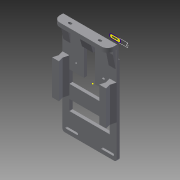
# Autodesk Inventor part: latte_d435_frame_s2new
Saved by Autodesk Inventor 2015 (Build 190159000, 159)
## iProperties
Created: 2021-11-17
Part Number: latte_d435_frame_s2new
Material: 常规
Document SubType Name: Modeling
Designer: chenhan
Density: 1 g/cm^3
Appearance: 默认
Author: chenhan
Autodesk Inventor part; units mm, degrees
ref_plane "YZ Plane" through (0, 0, 0) normal (1, 0, 0) x (0, 1, 0)
ref_plane "XZ Plane" through (0, 0, 0) normal (0, 1, 0) x (-1, 0, 0)
ref_plane "XY Plane" through (0, 0, 0) normal (0, 0, 1) x (1, 0, 0)
sketch "草图1" plane through (0, 0, 0) normal (0, 1, 0) x (-1, 0, 0)
  circle A0 centre (0, -42.5) radius 3.2
  circle A1 centre (0, -42.5) radius 1.6
  line L0 (63, 0) -> (-63, 0) projected
  circle A2 centre (19.7, 18.67) radius 1.6
  line L1 (0, -107.6) -> (0, 110.1) projected
  circle A3 centre (0, 42.5) radius 3.2
  circle A4 centre (0, 42.5) radius 1.6
  line L2 (-19.7, 18.67) -> (-19.7, -30.5269)
  line L3 (-19.7, -5.9284) -> (-19.7, -9.9284) construction
  line L4 (-20.95, -5.9284) -> (-20.95, -9.9284)
  line L5 (-18.45, -9.9284) -> (-18.45, -5.9284)
  arc A5 (-18.45, -5.9284) -> (-20.95, -5.9284) centre (-19.7, -5.9284) ccw
  arc A6 (-20.95, -9.9284) -> (-18.45, -9.9284) centre (-19.7, -9.9284) ccw
  line L6 (-22.2311, 18.67) -> (-17.1689, 18.67) construction
  line L7 (-18.7, 18.67) -> (-20.7, 18.67) construction
  line L8 (-18.7, 19.92) -> (-20.7, 19.92)
  line L9 (-20.7, 17.42) -> (-18.7, 17.42)
  arc A7 (-18.7, 17.42) -> (-18.7, 19.92) centre (-18.7, 18.67) ccw
  arc A8 (-20.7, 19.92) -> (-20.7, 17.42) centre (-20.7, 18.67) ccw
  line L10 (45, 79) -> (-45, 79)
  line L11 (-45, 79) -> (-45, 61.78)
  line L12 (-39, -76.5) -> (45, -76.5)
  line L13 (45, 61.78) -> (45, 79)
  line L14 (-39, 61.78) -> (-39, -76.5)
  line L15 (38, 73) -> (27.1169, 73)
  line L16 (39, 61.78) -> (45, 61.78)
  line L17 (-39, 61.78) -> (-45, 61.78)
  line L18 (37.25, 73) -> (27.25, 73) construction
  line L19 (37.25, 74.65) -> (27.25, 74.65)
  line L20 (27.25, 71.35) -> (37.25, 71.35)
  arc A9 (37.25, 71.35) -> (37.25, 74.65) centre (37.25, 73) ccw
  arc A10 (27.25, 74.65) -> (27.25, 71.35) centre (27.25, 73) ccw
  line L21 (34, -69.5) -> (18, -69.5) construction
  line L22 (34, -68) -> (18, -68)
  line L23 (18, -71) -> (34, -71)
  arc A11 (34, -71) -> (34, -68) centre (34, -69.5) ccw
  arc A12 (18, -68) -> (18, -71) centre (18, -69.5) ccw
  line L24 (-38, 73) -> (-27.1169, 73)
  line L25 (-37.25, 73) -> (-27.25, 73) construction
  line L26 (-37.25, 74.65) -> (-27.25, 74.65)
  line L27 (-27.25, 71.35) -> (-37.25, 71.35)
  arc A13 (-37.25, 74.65) -> (-37.25, 71.35) centre (-37.25, 73) ccw
  arc A14 (-27.25, 71.35) -> (-27.25, 74.65) centre (-27.25, 73) ccw
  line L28 (-34, -69.5) -> (-18, -69.5) construction
  line L29 (-34, -68) -> (-18, -68)
  line L30 (-18, -71) -> (-34, -71)
  arc A15 (-34, -68) -> (-34, -71) centre (-34, -69.5) ccw
  arc A16 (-18, -71) -> (-18, -68) centre (-18, -69.5) ccw
  line L31 (39, -27) -> (29, -27)
  line L32 (29, -27) -> (29, 23)
  line L33 (29, 23) -> (39, 23)
  line L34 (39, -27) -> (39, -27)
  line L35 (39, -27) -> (39, 31.5)
  line L36 (39, 31.5) -> (38.6344, 31.5)
  line L37 (39, 61.78) -> (39, 23)
  line L38 (39, -27) -> (39, -76.5)
  line L39 (39, -27) -> (29, -27)
  line L40 (29, -27) -> (29, 23)
  line L41 (29, 23) -> (39, 23)
  line L42 (39, 23) -> (39, -27)
  point P0 (0, 0)
  point P1 (-19.7, -7.9284)
  point P2 (32.25, 73)
  point P3 (26, -69.5)
  point P4 (-32.25, 73)
  point P5 (-26, -69.5)
  dimension "d0" = 6.4
  dimension "d1" = 3.2
  dimension "d2" = 42.5
  dimension "d7" = 3.2
  dimension "d8" = 19.7
  dimension "d9" = 18.67
  dimension "d10" = 4
  dimension "d14" = 2
  dimension "d15" = 2.5
  dimension "d16" = 39.4
  dimension "d18" = 90
  dimension "d20" = 45
  dimension "d23" = 3.3
  dimension "d24" = 32.25
  dimension "d25" = 10
  dimension "d27" = 16
  dimension "d28" = 3
  dimension "d30" = 26
  dimension "d56" = 106
  dimension "d57" = 50
  dimension "d67" = 10
  dimension "d85" = 2.5
  dimension "d86" = 4.35
  dimension "d127" = 79
  constraints: 95 end point, 24 point on circle, 19 symmetric about line, 17 centre point, 16 tangent, 10 parallel, 8 horizontal, 8 point on line, 7 perpendicular, 6 midpoint, 3 coincident, 2 vertical, 1 collinear, 6 other
  measures "d0" diameter of A0
  measures "d1" diameter of A1
  measures "d2" distance of point (0, 0) A0.centre
  measures "d7" diameter of A2
  measures "d8" horizontal distance of point (0, 0) A2.centre
  measures "d9" distance from line of L0 A2.centre
  measures "d10" distance of L3.start L3.end
  measures "d14" distance of L7.start L7.end
  measures "d15" diameter of A8
  measures "d16" distance from line of A2.centre L2
  measures "d18" distance of L10.start L10.end
  measures "d20" distance between parallel lines of L1 L13
  measures "d23" diameter of A10
  measures "d24" distance from line of L1 point (32.25, 73)
  measures "d25" distance of L18.end L18.start
  measures "d27" distance of L21.start L21.end
  measures "d28" diameter of A12
  measures "d30" distance from line of L1 point (26, -69.5)
  measures "d56" distance between parallel lines of L10 L31
  measures "d57" distance of L31.end L32.end
  measures "d67" distance between parallel lines of L35 L32
  measures "d85" distance between parallel lines of L5 L4
  measures "d86" distance between parallel lines of L10 L19
  measures "d127" distance between parallel lines of L10 L0
extrude "拉伸1" add sketch "草图1" along normal blind 4.5 contours A0 L1 L0 L32 L31 L38 L12 | A0 L1 L12 L14 L0 | L1 A3 L10 L13 L16 L37 L35 L33 L32 L0 | L0 L14 L17 L11 L10 L1 A3 | L32 L33 L35 L0 | L0 L35 L31 L32
fillet "圆角1" [suppressed]
fillet "圆角2" radius 3 2 edges at (39, 2.25, -76.5) (-39, 2.25, -76.5)
extrude "拉伸2" [suppressed]
sketch "草图2" plane through (0, 4.5, 0) normal (0, 1, 0) x (1, 0, 0)
  line L0 (27.25, -71.35) -> (37.25, -71.35) projected
  arc A0 (37.25, -74.65) -> (37.25, -71.35) centre (37.25, -73) ccw projected
  line L1 (37.25, -74.65) -> (27.25, -74.65) projected
  arc A1 (27.25, -71.35) -> (27.25, -74.65) centre (27.25, -73) ccw projected
  line L2 (37.25, -70) -> (27.25, -70)
  arc A2 (27.25, -70) -> (27.25, -76) centre (27.25, -73) ccw
  line L3 (27.25, -76) -> (37.25, -76)
  arc A3 (37.25, -76) -> (37.25, -70) centre (37.25, -73) ccw
  point P0 (0, 0)
  dimension "d37" = 6
  constraints: 4 end point, 4 point on circle, 2 centre point, 3 other
  measures "d37" distance between parallel lines of L3 L2
sketch "草图3" plane through (0, 0, 0) normal (0, -1, 0) x (1, 0, 0)
  arc A0 (37.25, 71.35) -> (37.25, 74.65) centre (37.25, 73) ccw projected
  line L0 (37.25, 71.35) -> (27.25, 71.35) projected
  line L1 (27.25, 74.65) -> (37.25, 74.65) projected
  arc A1 (27.25, 74.65) -> (27.25, 71.35) centre (27.25, 73) ccw projected
  line L2 (27.25, 70.4) -> (37.25, 70.4)
  arc A2 (37.25, 70.4) -> (37.25, 75.6) centre (37.25, 73) ccw
  line L3 (37.25, 75.6) -> (27.25, 75.6)
  arc A3 (27.25, 75.6) -> (27.25, 70.4) centre (27.25, 73) ccw
  point P0 (0, 0)
  dimension "d40" = 5.2
  constraints: 4 end point, 4 point on circle, 2 centre point, 3 other
  measures "d40" distance between parallel lines of L2 L3
extrude "拉伸4" cut sketch "草图3" against normal blind 2
mirror "镜像1" about plane through (0, 0, 0) normal (1, 0, 0) of "拉伸4"
sketch "草图4" plane through (0, 4.5, 0) normal (0, 1, 0) x (1, 0, 0)
  line L0 (35, 66) -> (-35, 66)
  line L1 (-35, 66) -> (-35, 57)
  line L2 (-35, 57) -> (35, 57)
  line L3 (35, 57) -> (35, 66)
  line L4 (-18, 68) -> (-34, 68) projected
  line L5 (7.5, 66) -> (-7.5, 66)
  line L6 (-7.5, 66) -> (-7.5, 57)
  line L7 (-7.5, 57) -> (7.5, 57)
  line L8 (7.5, 57) -> (7.5, 66)
  point P0 (0, 0)
  dimension "d43" = 70
  dimension "d44" = 9
  dimension "d45" = 35
  dimension "d46" = 2
  dimension "d47" = 15
  dimension "d48" = 7.5
  constraints: 16 end point, 4 parallel, 2 horizontal, 2 perpendicular, 2 point on line
  measures "d43" distance of L1.end L2.end
  measures "d44" distance of L2.end L0.start
  measures "d45" distance from line of L1 point (0, 0)
  measures "d46" distance between parallel lines of L0 L4
  measures "d47" distance between parallel lines of L8 L6
  measures "d48" distance from line of point (0, 0) L8
extrude "拉伸5" cut sketch "草图4" against normal blind 2.5 contours L3 L2 L8 L0 | L6 L2 L1 L0
sketch "草图5" plane through (0, 4.5, 0) normal (0, 1, 0) x (1, 0, 0)
  line L0 (18.45, 5.9284) -> (18.45, 9.9284) projected
  arc A0 (20.95, 9.9284) -> (18.45, 9.9284) centre (19.7, 9.9284) ccw projected
  line L1 (20.95, 9.9284) -> (20.95, 5.9284) projected
  arc A1 (18.45, 5.9284) -> (20.95, 5.9284) centre (19.7, 5.9284) ccw projected
  arc A2 (20.7, -19.92) -> (20.7, -17.42) centre (20.7, -18.67) ccw projected
  line L2 (20.7, -19.92) -> (18.7, -19.92) projected
  arc A3 (18.7, -17.42) -> (18.7, -19.92) centre (18.7, -18.67) ccw projected
  line L3 (18.7, -17.42) -> (20.7, -17.42) projected
  circle A4 centre (-19.7, -18.67) radius 1.6 projected
  line L4 (16.95, 9.9284) -> (16.95, 5.9284)
  arc A5 (16.95, 5.9284) -> (22.45, 5.9284) centre (19.7, 5.9284) ccw
  line L5 (22.45, 5.9284) -> (22.45, 9.9284)
  arc A6 (22.45, 9.9284) -> (16.95, 9.9284) centre (19.7, 9.9284) ccw
  line L6 (18.7, -21.42) -> (20.7, -21.42)
  arc A7 (20.7, -21.42) -> (20.7, -15.92) centre (20.7, -18.67) ccw
  line L7 (20.7, -15.92) -> (18.7, -15.92)
  arc A8 (18.7, -15.92) -> (18.7, -21.42) centre (18.7, -18.67) ccw
  circle A9 centre (-19.7, -18.67) radius 3
  point P0 (0, 0)
  dimension "d51" = 1.5
  dimension "d52" = 1.5
  dimension "d53" = 6
  constraints: 8 end point, 8 point on circle, 5 centre point, 6 other
  measures "d51" distance between parallel lines of L0 L4
  measures "d52" distance between parallel lines of L6 L2
  measures "d53" diameter of A9
extrude "拉伸6" [suppressed]
extrude "拉伸9" [suppressed]
sketch "草图7" plane through (-41, 4.5, 31.5) normal (0, 0, 1) x (1, 0, 0)
  point P0 (41, -4.5)
sketch "草图8" plane through (-39, 4.5, -18.5) normal (0, 0, -1) x (-1, 0, 0)
  line L0 (0, 0) -> (0, -4.5) projected
  line L1 (-8, -4.5) -> (0, -4.5) projected
  line L2 (-8, -4.5) -> (-8, -19.5) projected
  line L3 (2, -19.5) -> (-8, -19.5) projected
  line L4 (2, -19.5) -> (2, 0) projected
  line L5 (0, 0) -> (2, 0) projected
  line L6 (-8, -19.5) -> (2, -19.5) projected
  line L7 (-8, -19.5) -> (-6, -12)
  line L8 (-6, -12) -> (-8, -4.5)
  line L9 (3, -4.5) -> (-81, -4.5) projected
  line L10 (2, -19.5) -> (0, -12)
  line L11 (0, -12) -> (2, -4.5)
  line L12 (2, -19.5) -> (2, 0) projected
  point P0 (-39, -4.5)
  dimension "d71" = 2
  dimension "d72" = 7.5
  dimension "d73" = 2
  dimension "d74" = 7.5
  constraints: 8 end point, 2 point on line
  measures "d71" distance from line of L2 L7.end
  measures "d72" distance from line of L3 L7.end
  measures "d73" distance from line of L4 L10.end
  measures "d74" distance from line of L3 L10.end
extrude "拉伸10" [suppressed]
mirror "镜像4" [suppressed]
extrude "拉伸11" add sketch "草图1" against normal blind 15 contours L32 L33 L35 L0 | L0 L35 L31 L32
sketch "草图9" plane through (-29, 0, -27) normal (0, 0, -1) x (-1, 0, 0)
  line L0 (0, 0) -> (10, 0) projected
  line L1 (0, 0) -> (0, -15) projected
  line L2 (10, -15) -> (0, -15) projected
  line L3 (10, 0) -> (10, -15) projected
  line L4 (0, -15) -> (2, -7.5)
  line L5 (2, -7.5) -> (0, 0)
  line L6 (10, 0) -> (8, -7.5)
  line L7 (8, -7.5) -> (10, -15)
  point P0 (-29, 0)
  dimension "d79" = 2
  dimension "d80" = 7.5
  dimension "d81" = 7.5
  dimension "d82" = 2
  constraints: 8 end point
  measures "d79" distance from line of L1 L4.end
  measures "d80" distance from line of L2 L4.end
  measures "d81" distance from line of L2 L6.end
  measures "d82" distance from line of L3 L6.end
extrude "拉伸12" cut sketch "草图9" against normal through all contours L5 L4 L1 | L3 L7 L6
mirror "镜像5" about plane through (0, 0, 0) normal (1, 0, 0) of "拉伸12", "拉伸11"
sketch "草图10" plane through (-45, 0, 79) normal (0, 0, 1) x (1, 0, 0)
  line L0 (0, 0) -> (90, 0) projected
  line L1 (90, 0) -> (90, 4.5) projected
  line L2 (0, 4.5) -> (90, 4.5) projected
  line L3 (0, 0) -> (0, 4.5) projected
  point P0 (45, 0)
extrude "拉伸13" add sketch "草图10" along normal blind 2
sketch "草图11" plane through (0, 4.5, 0) normal (0, 1, 0) x (1, 0, 0)
  line L0 (7.5, 57) -> (7.5, 66) projected
  line L1 (35, 57) -> (7.5, 57) projected
  line L2 (35, 66) -> (35, 57) projected
  line L3 (7.5, 66) -> (35, 66) projected
  point P0 (0, 0)
sketch "草图12" plane through (0, 4.5, 0) normal (0, 1, 0) x (1, 0, 0)
  line L0 (45, -61.78) -> (45, -81) projected
  line L1 (-45, -81) -> (45, -81)
  line L2 (45, -81) -> (45, -70)
  line L3 (45, -70) -> (-45, -70)
  line L4 (-45, -70) -> (-45, -81)
  circle A0 centre (0, -42.5) radius 3.2 projected
  point P0 (0, 0)
  dimension "d90" = 11
  constraints: 8 end point, 2 parallel, 1 horizontal, 1 perpendicular, 1 point on line
  measures "d90" distance between parallel lines of L1 L3
extrude "拉伸14" cut sketch "草图12" against normal blind 10 contours L0 L1 L4 L3
sketch "草图13" plane through (0, 4.5, 0) normal (0, 1, 0) x (1, 0, 0)
  line L0 (-45, -70) -> (-39, -70)
  line L1 (-39, -70) -> (-39, -61.78)
  line L2 (-39, -61.78) -> (-45, -61.78)
  line L3 (-45, -61.78) -> (-45, -70)
  line L4 (-45, -70) -> (45, -70) projected
  line L5 (45, -61.78) -> (39, -61.78)
  line L6 (39, -61.78) -> (39, -70)
  line L7 (39, -70) -> (45, -70)
  line L8 (45, -70) -> (45, -61.78)
  point P0 (0, 0)
  constraints: 16 end point, 4 parallel, 2 horizontal, 2 perpendicular, 2 point on line
extrude "拉伸15" cut sketch "草图13" against normal blind 10
sketch "草图14" plane through (0, 0, 0) normal (0, -1, 0) x (1, 0, 0)
  line L0 (-39, -73.5) -> (-39, 70) projected
  line L1 (39, 70) -> (-39, 70)
  line L2 (-39, 70) -> (-39, 64)
  line L3 (-39, 64) -> (39, 64)
  line L4 (39, 64) -> (39, 70)
  point P0 (0, 0)
  dimension "d95" = 6
  constraints: 8 end point, 2 parallel, 1 horizontal, 1 perpendicular, 1 point on line
  measures "d95" distance between parallel lines of L1 L3
extrude "拉伸16" add sketch "草图14" along normal blind 13
sketch "草图15" plane through (-0.5568, 0, 64) normal (0, 0, -1) x (-1, 0, 0)
  line L0 (22.0432, -8) -> (20.0432, -8)
  line L1 (20.0432, -4.8) -> (22.0432, -4.8)
  arc A0 (22.0432, -8) -> (22.0432, -4.8) centre (22.0432, -6.4) ccw
  arc A1 (20.0432, -4.8) -> (20.0432, -8) centre (20.0432, -6.4) ccw
  line L2 (20.0432, -9.5) -> (22.0432, -9.5)
  arc A2 (22.0432, -9.5) -> (22.0432, -3.3) centre (22.0432, -6.4) ccw
  line L3 (22.0432, -3.3) -> (20.0432, -3.3)
  arc A3 (20.0432, -3.3) -> (20.0432, -9.5) centre (20.0432, -6.4) ccw
  line L4 (-0.5568, -18.9) -> (-0.5568, 8.4) projected
  line L5 (38.4432, -13) -> (-39.5568, -13) projected
  line L6 (-23.1568, -8) -> (-21.1568, -8)
  line L7 (-21.1568, -4.8) -> (-23.1568, -4.8)
  arc A4 (-23.1568, -4.8) -> (-23.1568, -8) centre (-23.1568, -6.4) ccw
  arc A5 (-21.1568, -8) -> (-21.1568, -4.8) centre (-21.1568, -6.4) ccw
  line L8 (-21.1568, -9.5) -> (-23.1568, -9.5)
  arc A6 (-23.1568, -3.3) -> (-23.1568, -9.5) centre (-23.1568, -6.4) ccw
  line L9 (-23.1568, -3.3) -> (-21.1568, -3.3)
  arc A7 (-21.1568, -9.5) -> (-21.1568, -3.3) centre (-21.1568, -6.4) ccw
  line L10 (-39.5568, -13) -> (38.4432, -13)
  point P0 (-0.5568, 0)
  point P1 (35.25, 0)
  dimension "d100" = 1.6
  dimension "d102" = 6.2
  dimension "d103" = 22.6
  dimension "d104" = 1.6
  dimension "d105" = 3.1
  dimension "d106" = 3.5
  dimension "d107" = 2
  constraints: 18 end point, 16 point on circle, 12 symmetric about line, 8 centre point, 1 perpendicular, 7 other
  measures "d100" radius of A0
  measures "d102" distance between parallel lines of L2 L3
  measures "d103" distance from line of L4 A0.centre
  measures "d104" radius of A1
  measures "d105" radius of A3
  measures "d106" distance between parallel lines of L5 L2
  measures "d107" distance of A0.centre A1.centre
extrude "拉伸17" cut sketch "草图15" against normal blind 2
extrude "拉伸18" cut sketch "草图15" against normal through all contours L0 A1 L1 A0 | A4 L7 A5 L6
sketch "草图16" plane through (0, 4.5, 0) normal (0, 1, 0) x (1, 0, 0)
  line L0 (39, -70) -> (-39, -70) projected
  line L1 (-8, -38) -> (8, -38)
  line L2 (8, -38) -> (8, -70)
  line L3 (8, -70) -> (-8, -70)
  line L4 (-8, -70) -> (-8, -38)
  circle A0 centre (0, -42.5) radius 1.6 projected
  point P0 (0, 0)
  dimension "d112" = 16
  dimension "d113" = 32
  dimension "d114" = 8
  constraints: 8 end point, 2 parallel, 1 horizontal, 1 perpendicular, 1 point on line
  measures "d112" distance between parallel lines of L2 L4
  measures "d113" distance of L3.end L1.start
  measures "d114" distance from line of A0.centre L4
extrude "拉伸19" add sketch "草图16" against normal blind 12 contours L0 L4 L1 L2 | A0
chamfer "倒角1" distance 25 distance2 7 1 edges at (0, -7.5, 38) measured on face at (-2.6667, -7.5, 46.6667)
fillet "圆角3" radius 9 2 edges at (39, -13, 67) (-39, -13, 67)
sketch "草图17" plane through (0, 4.5, 0) normal (0, 1, 0) x (1, 0, 0)
  circle A0 centre (0, 42.5) radius 3.2 projected
  line L0 (29, 46.6572) -> (-29, 46.6572)
  line L1 (-29, 46.6572) -> (-29, 31.6572)
  line L2 (-29, 31.6572) -> (29, 31.6572)
  line L3 (29, 31.6572) -> (29, 46.6572)
  line L4 (39, -70) -> (39, 73.5) projected
  line L5 (-39, 73.5) -> (-39, -70) projected
  line L6 (-31, 27) -> (-31, -23) projected
  line L7 (14.0388, 12.562) -> (-31, 12.562)
  line L8 (-31, 12.562) -> (-31, -5.438)
  line L9 (-31, -5.438) -> (14.0388, -5.438)
  line L10 (14.0388, -5.438) -> (14.0388, 12.562)
  line L11 (-29, 27) -> (-29, -23) projected
  line L12 (-29, 12.562) -> (-29, -5.438)
  line L13 (8, -46.1765) -> (-8, -46.1765)
  line L14 (-8, -46.1765) -> (-8, -5.438)
  line L15 (-8, -5.438) -> (8, -5.438)
  line L16 (8, -5.438) -> (8, -46.1765)
  point P0 (0, 0)
  dimension "d121" = 10
  dimension "d122" = 10
  dimension "d123" = 15
  dimension "d124" = 18
  dimension "d125" = 31
  dimension "d126" = 31
  constraints: 26 end point, 6 parallel, 6 point on line, 3 horizontal, 3 perpendicular
  measures "d121" distance between parallel lines of L4 L3
  measures "d122" distance between parallel lines of L5 L1
  measures "d123" distance between parallel lines of L2 L0
  measures "d124" distance between parallel lines of L9 L7
  measures "d125" distance between parallel lines of L16 L4
  measures "d126" distance between parallel lines of L5 L14
extrude "拉伸20" cut sketch "草图17" against normal through all contours L3 L2 L1 L0 | L7 L10 L9 L11 | L9 L16 L13 L14
sketch "草图18" plane through (-39, 0, -73.5) normal (-1, 0, 0) x (0, 0, 1)
  line L0 (143.5, 4.5) -> (0, 4.5) projected
  line L1 (143.5, 4.5) -> (143.5, -4) projected
  line L2 (123.5, 4.5) -> (143.5, 4.5)
  line L3 (143.5, 4.5) -> (143.5, 3)
  line L4 (143.5, 3) -> (123.5, 3)
  line L5 (123.5, 3) -> (123.5, 4.5)
  point P0 (73.5, 0)
  dimension "d130" = 1.5
  dimension "d131" = 20
  constraints: 8 end point, 2 parallel, 2 point on line, 1 horizontal, 1 perpendicular
  measures "d130" distance of L4.end L2.start
  measures "d131" distance of L3.end L4.end
extrude "拉伸21" cut sketch "草图18" against normal through all
sketch "草图19" plane through (-8, 0, 64) normal (0, 0, -1) x (-1, 0, 0)
  line L0 (0, 0) -> (31, 0) projected
  line L1 (19.726, 0) -> (29.726, 0)
  line L2 (29.726, 0) -> (29.726, -4)
  line L3 (29.726, -4) -> (19.726, -4)
  line L4 (19.726, -4) -> (19.726, 0)
  point P0 (-8, 0)
  dimension "d134" = 10
  dimension "d135" = 4
  constraints: 8 end point, 2 parallel, 1 horizontal, 1 perpendicular, 1 point on line
  measures "d134" distance of L2.end L3.end
  measures "d135" distance of L1.end L2.end
extrude "拉伸22" add sketch "草图19" along normal blind 25
chamfer "倒角2" distance 4 distance2 20 1 edges at (-32.726, -4, 39) measured on face at (-31.0594, -1.3333, 39)
mirror "镜像6" about plane through (0, 0, 0) normal (1, 0, 0) of "拉伸22", "倒角2"
chamfer "倒角3" distance 2 angle 45 1 edges at (0, 3, 70)
